Autodesk Inventor part; units mm, degrees
(part 2 of 2)
  arc A370 (45.3875, -111.275) -> (45.8875, -111.775) centre (45.8875, -111.275) ccw
  arc A371 (58.8875, -111.775) -> (59.3875, -111.275) centre (58.8875, -111.275) ccw
  line L372 (69.7, -97.775) -> (82.7, -97.775)
  line L373 (69.7, -111.775) -> (82.7, -111.775)
  line L374 (69.2, -98.275) -> (69.2, -111.275)
  line L375 (83.2, -98.275) -> (83.2, -111.275)
  arc A372 (69.7, -97.775) -> (69.2, -98.275) centre (69.7, -98.275) ccw
  arc A373 (83.2, -98.275) -> (82.7, -97.775) centre (82.7, -98.275) ccw
  arc A374 (69.2, -111.275) -> (69.7, -111.775) centre (69.7, -111.275) ccw
  arc A375 (82.7, -111.775) -> (83.2, -111.275) centre (82.7, -111.275) ccw
  line L376 (93.5125, -97.775) -> (106.5125, -97.775)
  line L377 (93.5125, -111.775) -> (106.5125, -111.775)
  line L378 (93.0125, -98.275) -> (93.0125, -111.275)
  line L379 (107.0125, -98.275) -> (107.0125, -111.275)
  arc A376 (93.5125, -97.775) -> (93.0125, -98.275) centre (93.5125, -98.275) ccw
  arc A377 (107.0125, -98.275) -> (106.5125, -97.775) centre (106.5125, -98.275) ccw
  arc A378 (93.0125, -111.275) -> (93.5125, -111.775) centre (93.5125, -111.275) ccw
  arc A379 (106.5125, -111.775) -> (107.0125, -111.275) centre (106.5125, -111.275) ccw
  line L380 (167.3313, -97.775) -> (180.3313, -97.775)
  line L381 (167.3313, -111.775) -> (180.3313, -111.775)
  line L382 (166.8313, -98.275) -> (166.8313, -111.275)
  line L383 (180.8313, -98.275) -> (180.8313, -111.275)
  arc A380 (167.3313, -97.775) -> (166.8313, -98.275) centre (167.3313, -98.275) ccw
  arc A381 (180.8313, -98.275) -> (180.3313, -97.775) centre (180.3313, -98.275) ccw
  arc A382 (166.8313, -111.275) -> (167.3313, -111.775) centre (167.3313, -111.275) ccw
  arc A383 (180.3313, -111.775) -> (180.8313, -111.275) centre (180.3313, -111.275) ccw
  line L384 (220.9563, -98.775) -> (226.7063, -98.775)
  line L385 (220.9563, -112.775) -> (226.7063, -112.775)
  line L386 (220.4563, -99.275) -> (220.4563, -112.275)
  line L387 (227.2063, -99.275) -> (227.2063, -112.275)
  arc A384 (220.9563, -98.775) -> (220.4563, -99.275) centre (220.9563, -99.275) ccw
  arc A385 (227.2063, -99.275) -> (226.7063, -98.775) centre (226.7063, -99.275) ccw
  arc A386 (220.4563, -112.275) -> (220.9563, -112.775) centre (220.9563, -112.275) ccw
  arc A387 (226.7063, -112.775) -> (227.2063, -112.275) centre (226.7063, -112.275) ccw
  line L388 (120.9562, -98.775) -> (126.7063, -98.775)
  line L389 (120.9562, -112.775) -> (126.7063, -112.775)
  line L390 (120.4563, -99.275) -> (120.4563, -112.275)
  line L391 (127.2062, -99.275) -> (127.2062, -112.275)
  arc A388 (120.9562, -98.775) -> (120.4563, -99.275) centre (120.9562, -99.275) ccw
  arc A389 (127.2062, -99.275) -> (126.7063, -98.775) centre (126.7063, -99.275) ccw
  arc A390 (120.4563, -112.275) -> (120.9562, -112.775) centre (120.9562, -112.275) ccw
  arc A391 (126.7063, -112.775) -> (127.2062, -112.275) centre (126.7063, -112.275) ccw
  line L392 (238.7688, -97.775) -> (251.7687, -97.775)
  line L393 (238.7688, -111.775) -> (251.7687, -111.775)
  line L394 (238.2688, -98.275) -> (238.2688, -111.275)
  line L395 (252.2688, -98.275) -> (252.2688, -111.275)
  arc A392 (238.7688, -97.775) -> (238.2688, -98.275) centre (238.7688, -98.275) ccw
  arc A393 (252.2688, -98.275) -> (251.7687, -97.775) centre (251.7687, -98.275) ccw
  arc A394 (238.2688, -111.275) -> (238.7688, -111.775) centre (238.7688, -111.275) ccw
  arc A395 (251.7687, -111.775) -> (252.2688, -111.275) centre (251.7687, -111.275) ccw
  line L396 (264.9625, -97.775) -> (277.9625, -97.775)
  line L397 (264.9625, -111.775) -> (277.9625, -111.775)
  line L398 (264.4625, -98.275) -> (264.4625, -111.275)
  line L399 (278.4625, -98.275) -> (278.4625, -111.275)
  arc A396 (264.9625, -97.775) -> (264.4625, -98.275) centre (264.9625, -98.275) ccw
  arc A397 (278.4625, -98.275) -> (277.9625, -97.775) centre (277.9625, -98.275) ccw
  arc A398 (264.4625, -111.275) -> (264.9625, -111.775) centre (264.9625, -111.275) ccw
  arc A399 (277.9625, -111.775) -> (278.4625, -111.275) centre (277.9625, -111.275) ccw
  line L400 (288.775, -97.775) -> (301.775, -97.775)
  line L401 (288.775, -111.775) -> (301.775, -111.775)
  line L402 (288.275, -98.275) -> (288.275, -111.275)
  line L403 (302.275, -98.275) -> (302.275, -111.275)
  arc A400 (288.775, -97.775) -> (288.275, -98.275) centre (288.775, -98.275) ccw
  arc A401 (302.275, -98.275) -> (301.775, -97.775) centre (301.775, -98.275) ccw
  arc A402 (288.275, -111.275) -> (288.775, -111.775) centre (288.775, -111.275) ccw
  arc A403 (301.775, -111.775) -> (302.275, -111.275) centre (301.775, -111.275) ccw
  line L404 (307.825, -97.775) -> (320.825, -97.775)
  line L405 (307.825, -111.775) -> (320.825, -111.775)
  line L406 (307.325, -98.275) -> (307.325, -111.275)
  line L407 (321.325, -98.275) -> (321.325, -111.275)
  arc A404 (307.825, -97.775) -> (307.325, -98.275) centre (307.825, -98.275) ccw
  arc A405 (321.325, -98.275) -> (320.825, -97.775) centre (320.825, -98.275) ccw
  arc A406 (307.325, -111.275) -> (307.825, -111.775) centre (307.825, -111.275) ccw
  arc A407 (320.825, -111.775) -> (321.325, -111.275) centre (320.825, -111.275) ccw
  line L408 (326.875, -97.775) -> (339.875, -97.775)
  line L409 (326.875, -111.775) -> (339.875, -111.775)
  line L410 (326.375, -98.275) -> (326.375, -111.275)
  line L411 (340.375, -98.275) -> (340.375, -111.275)
  arc A408 (326.875, -97.775) -> (326.375, -98.275) centre (326.875, -98.275) ccw
  arc A409 (340.375, -98.275) -> (339.875, -97.775) centre (339.875, -98.275) ccw
  arc A410 (326.375, -111.275) -> (326.875, -111.775) centre (326.875, -111.275) ccw
  arc A411 (339.875, -111.775) -> (340.375, -111.275) centre (339.875, -111.275) ccw
  line L412 (0, 0) -> (342.9, 0)
  line L413 (0, -114.3) -> (342.9, -114.3)
  line L414 (0, 0) -> (0, -114.3)
  line L415 (342.9, 0) -> (342.9, -114.3)
  line L416 (342.9, 0) -> (0, 0)
  line L417 (0, 0) -> (0, -114.3)
  line L418 (0, -114.3) -> (342.9, -114.3)
  line L419 (342.9, -114.3) -> (342.9, 0)
  line L420 (2.525, -16.525) -> (16.525, -16.525)
  line L421 (16.525, -16.525) -> (16.525, -2.525)
  line L422 (16.525, -2.525) -> (2.525, -2.525)
  line L423 (2.525, -2.525) -> (2.525, -16.525)
  line L424 (2.525, -16.525) -> (16.525, -2.525) construction
  line L425 (16.525, -16.525) -> (2.525, -2.525) construction
  point P0 (207.3125, -73.175)
  point P1 (207.3125, -60.175)
  point P2 (226.3625, -73.175)
  point P3 (226.3625, -60.175)
  point P4 (278.4625, -60.175)
  point P5 (278.4625, -73.175)
  point P6 (16.525, -79.225)
  point P7 (16.525, -92.225)
  point P8 (16.025, -92.725)
  point P9 (3.025, -92.725)
  point P10 (35.075, -92.725)
  point P11 (22.075, -92.725)
  point P12 (66.0312, -92.725)
  point P13 (53.0313, -92.725)
  point P14 (96.9875, -92.725)
  point P15 (83.9875, -92.725)
  point P16 (83.4875, -92.225)
  point P17 (83.4875, -79.225)
  point P18 (116.0375, -92.725)
  point P19 (103.0375, -92.725)
  point P20 (135.0875, -92.725)
  point P21 (122.0875, -92.725)
  point P22 (154.6375, -79.225)
  point P23 (154.6375, -92.225)
  point P24 (154.1375, -92.725)
  point P25 (141.1375, -92.725)
  point P26 (173.1875, -92.725)
  point P27 (160.1875, -92.725)
  point P28 (192.2375, -92.725)
  point P29 (179.2375, -92.725)
  point P30 (211.2875, -92.725)
  point P31 (198.2875, -92.725)
  point P32 (197.7875, -92.225)
  point P33 (197.7875, -79.225)
  point P34 (230.3375, -92.725)
  point P35 (217.3375, -92.725)
  point P36 (216.8375, -92.225)
  point P37 (216.8375, -79.225)
  point P38 (249.3875, -92.725)
  point P39 (236.3875, -92.725)
  point P40 (268.4375, -92.725)
  point P41 (255.4375, -92.725)
  point P42 (295.1313, -79.225)
  point P43 (295.1313, -92.225)
  point P44 (294.6313, -92.725)
  point P45 (281.6313, -92.725)
  point P46 (320.825, -92.725)
  point P47 (307.825, -92.725)
  point P48 (307.325, -92.225)
  point P49 (307.325, -79.225)
  point P50 (339.875, -92.725)
  point P51 (326.875, -92.725)
  point P52 (3.025, -97.775)
  point P53 (16.025, -97.775)
  point P54 (16.525, -98.275)
  point P55 (16.525, -111.275)
  point P56 (22.075, -97.775)
  point P57 (35.075, -97.775)
  point P58 (45.8875, -97.775)
  point P59 (58.8875, -97.775)
  point P60 (69.7, -97.775)
  point P61 (82.7, -97.775)
  point P62 (83.2, -98.275)
  point P63 (83.2, -111.275)
  point P64 (93.5125, -97.775)
  point P65 (106.5125, -97.775)
  point P66 (93.0125, -111.275)
  point P67 (93.0125, -98.275)
  point P68 (167.3313, -97.775)
  point P69 (180.3313, -97.775)
  point P70 (127.2063, -99.275)
  point P71 (127.2063, -112.275)
  point P72 (120.4562, -112.275)
  point P73 (120.4562, -99.275)
  point P74 (238.7688, -97.775)
  point P75 (251.7687, -97.775)
  point P76 (264.9625, -97.775)
  point P77 (277.9625, -97.775)
  point P78 (278.4625, -98.275)
  point P79 (278.4625, -111.275)
  point P80 (288.775, -97.775)
  point P81 (301.775, -97.775)
  point P82 (307.825, -97.775)
  point P83 (320.825, -97.775)
  point P84 (307.325, -111.275)
  point P85 (307.325, -98.275)
  point P86 (326.875, -97.775)
  point P87 (339.875, -97.775)
  point P88 (263.675, -16.525)
  point P89 (250.675, -16.525)
  point P90 (282.725, -16.525)
  point P91 (269.725, -16.525)
  point P92 (301.775, -16.525)
  point P93 (288.775, -16.525)
  point P94 (320.825, -16.525)
  point P95 (307.825, -16.525)
  point P96 (307.325, -16.025)
  point P97 (307.325, -3.025)
  point P98 (339.875, -16.525)
  point P99 (326.875, -16.525)
  point P100 (16.525, -22.075)
  point P101 (16.525, -35.075)
  point P102 (92.725, -22.075)
  point P103 (92.725, -35.075)
  point P104 (97.775, -35.075)
  point P105 (97.775, -22.075)
  point P106 (207.025, -22.075)
  point P107 (207.025, -35.075)
  point P108 (313.863, -22.575)
  point P109 (319.613, -22.575)
  point P110 (289.987, -22.575)
  point P111 (295.737, -22.575)
  point P112 (16.525, -41.125)
  point P113 (16.525, -54.125)
  point P114 (83.2, -41.125)
  point P115 (83.2, -54.125)
  point P116 (88.25, -54.125)
  point P117 (88.25, -41.125)
  point P118 (197.5, -41.125)
  point P119 (197.5, -54.125)
  point P120 (216.55, -41.125)
  point P121 (216.55, -54.125)
  point P122 (316.5625, -41.125)
  point P123 (316.5625, -54.125)
  point P124 (16.525, -60.175)
  point P125 (16.525, -73.175)
  point P126 (47.7688, -73.175)
  point P127 (47.7688, -60.175)
  point P128 (87.9625, -60.175)
  point P129 (87.9625, -73.175)
  point P130 (93.0125, -73.175)
  point P131 (93.0125, -60.175)
  point P132 (92.725, -3.025)
  point P133 (92.725, -16.025)
  point P134 (92.225, -16.525)
  point P135 (79.225, -16.525)
  point P136 (16.525, -3.025)
  point P137 (16.525, -16.025)
  point P138 (16.025, -16.525)
  point P139 (3.025, -16.525)
  point P140 (155.425, -16.525)
  point P141 (97.775, -3.025)
  point P142 (187.475, -16.525)
  point P143 (174.475, -16.525)
  point P144 (207.025, -3.025)
  point P145 (207.025, -16.025)
  point P146 (225.575, -16.525)
  point P147 (54.125, -16.525)
  point P148 (41.125, -16.525)
  point P149 (130.325, -16.525)
  point P150 (117.325, -16.525)
  point P151 (9.525, -9.525)
  constraints: 852 end point, 824 point on circle, 412 centre point, 4 parallel, 2 horizontal, 2 midpoint, 2 perpendicular
extrude "Plate2" add sketch "Sketch1" along normal blind 0.5 contours L0 A1 L3 A3 L1 A2 L2 A0 | A0 L423 L422 | L422 L421 A1 | A2 L420 L423 | L421 L420 A3 | L4 A5 L7 A7 L5 A6 L6 A4 | L8 A9 L11 A11 L9 A10 L10 A8 | L12 A13 L15 A15 L13 A14 L14 A12 | L16 A17 L19 A19 L17 A18 L18 A16 | L20 A21 L23 A23 L21 A22 L22 A20 | L24 A25 L27 A27 L25 A26 L26 A24 | L28 A29 L31 A31 L29 A30 L30 A28 | L32 A33 L35 A35 L33 A34 L34 A32 | L36 A37 L39 A39 L37 A38 L38 A36 | L40 A41 L43 A43 L41 A42 L42 A40 | L44 A45 L47 A47 L45 A46 L46 A44 | L48 A49 L51 A51 L49 A50 L50 A48 | L52 A53 L55 A55 L53 A54 L54 A52 | L56 A57 L59 A59 L57 A58 L58 A56 | L60 A61 L63 A63 L61 A62 L62 A60 | L64 A65 L67 A67 L65 A66 L66 A64 | L68 A69 L71 A71 L69 A70 L70 A68 | L72 A73 L75 A75 L73 A74 L74 A72 | L76 A77 L79 A79 L77 A78 L78 A76 | L80 A81 L83 A83 L81 A82 L82 A80 | L84 A85 L87 A87 L85 A86 L86 A84 | L88 A89 L91 A91 L89 A90 L90 A88 | L92 A93 L95 A95 L93 A94 L94 A92 | L96 A97 L99 A99 L97 A98 L98 A96 | L100 A101 L103 A103 L101 A102 L102 A100 | L104 A105 L107 A107 L105 A106 L106 A104 | L108 A109 L111 A111 L109 A110 L110 A108 | L112 A113 L115 A115 L113 A114 L114 A112 | L116 A117 L119 A119 L117 A118 L118 A116 | L120 A121 L123 A123 L121 A122 L122 A120 | L124 A125 L127 A127 L125 A126 L126 A124 | L128 A129 L131 A131 L129 A130 L130 A128 | L132 A133 L135 A135 L133 A134 L134 A132 | L136 A137 L139 A139 L137 A138 L138 A136 | L140 A141 L143 A143 L141 A142 L142 A140 | L144 A145 L147 A147 L145 A146 L146 A144 | L148 A149 L151 A151 L149 A150 L150 A148 | L152 A153 L155 A155 L153 A154 L154 A152 | L156 A157 L159 A159 L157 A158 L158 A156 | L160 A161 L163 A163 L161 A162 L162 A160 | L164 A165 L167 A167 L165 A166 L166 A164 | L168 A169 L171 A171 L169 A170 L170 A168 | L172 A173 L175 A175 L173 A174 L174 A172 | L176 A177 L179 A179 L177 A178 L178 A176 | L180 A181 L183 A183 L181 A182 L182 A180 | L184 A185 L187 A187 L185 A186 L186 A184 | L188 A189 L191 A191 L189 A190 L190 A188 | L192 A193 L195 A195 L193 A194 L194 A192 | L196 A197 L199 A199 L197 A198 L198 A196 | L200 A201 L203 A203 L201 A202 L202 A200 | L204 A205 L207 A207 L205 A206 L206 A204 | L208 A209 L211 A211 L209 A210 L210 A208 | L212 A213 L215 A215 L213 A214 L214 A212 | L216 A217 L219 A219 L217 A218 L218 A216 | L220 A221 L223 A223 L221 A222 L222 A220 | L224 A225 L227 A227 L225 A226 L226 A224 | L228 A229 L231 A231 L229 A230 L230 A228 | L232 A233 L235 A235 L233 A234 L234 A232 | L236 A237 L239 A239 L237 A238 L238 A236 | L240 A241 L243 A243 L241 A242 L242 A240 | L244 A245 L247 A247 L245 A246 L246 A244 | L248 A249 L251 A251 L249 A250 L250 A248 | L252 A253 L255 A255 L253 A254 L254 A252 | L256 A257 L259 A259 L257 A258 L258 A256 | L260 A261 L263 A263 L261 A262 L262 A260 | L264 A265 L267 A267 L265 A266 L266 A264 | L268 A269 L271 A271 L269 A270 L270 A268 | L272 A273 L275 A275 L273 A274 L274 A272 | L276 A277 L279 A279 L277 A278 L278 A276 | L280 A281 L283 A283 L281 A282 L282 A280 | L284 A285 L287 A287 L285 A286 L286 A284 | L288 A289 L291 A291 L289 A290 L290 A288 | L292 A293 L295 A295 L293 A294 L294 A292 | L296 A297 L299 A299 L297 A298 L298 A296 | L300 A301 L303 A303 L301 A302 L302 A300 | L304 A305 L307 A307 L305 A306 L306 A304 | L308 A309 L311 A311 L309 A310 L310 A308 | L312 A313 L315 A315 L313 A314 L314 A312 | L316 A317 L319 A319 L317 A318 L318 A316 | L320 A321 L323 A323 L321 A322 L322 A320 | L324 A325 L327 A327 L325 A326 L326 A324 | L328 A329 L331 A331 L329 A330 L330 A328 | L332 A333 L335 A335 L333 A334 L334 A332 | L336 A337 L339 A339 L337 A338 L338 A336 | L340 A341 L343 A343 L341 A342 L342 A340 | L344 A345 L347 A347 L345 A346 L346 A344 | L348 A349 L351 A351 L349 A350 L350 A348 | L352 A353 L355 A355 L353 A354 L354 A352 | L356 A357 L359 A359 L357 A358 L358 A356 | L360 A361 L363 A363 L361 A362 L362 A360 | L364 A365 L367 A367 L365 A366 L366 A364 | L368 A369 L371 A371 L369 A370 L370 A368 | L372 A373 L375 A375 L373 A374 L374 A372 | L376 A377 L379 A379 L377 A378 L378 A376 | L380 A381 L383 A383 L381 A382 L382 A380 | L384 A385 L387 A387 L385 A386 L386 A384 | L388 A389 L391 A391 L389 A390 L390 A388 | L392 A393 L395 A395 L393 A394 L394 A392 | L396 A397 L399 A399 L397 A398 L398 A396 | L400 A401 L403 A403 L401 A402 L402 A400 | L404 A405 L407 A407 L405 A406 L406 A404 | L408 A409 L411 A411 L409 A410 L410 A408 | L412 L415 L413 L414
extrude "Cut1" cut sketch "Sketch1" along normal through all both and the other way through all contours L0 A1 L3 A3 L1 A2 L2 A0 | A0 L423 L422 | L422 L421 A1 | A2 L420 L423 | L421 L420 A3
equation "\"d16\" = Thickness"
equation "\"d15\" = Thickness"
equation "\"BendRadius\" = Thickness"
equation "\"BendReliefWidth\" = Thickness"
equation "\"BendReliefDepth\" = 0.5 * Thickness"
equation "\"CornerReliefSize\" = 4 * Thickness"
equation "\"MinimumRemnant\" = 2 * Thickness"
equation "\"TransitionRadius\" = BendRadius"
equation "\"JacobiRadiusSize\" = BendRadius"
equation "\"GapSize\" = Thickness"
equation "\"Thickness\" = 0.5"
body "Solid2"
